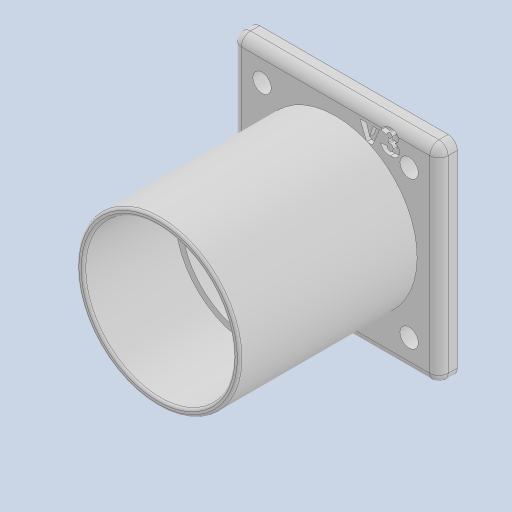
# Autodesk Inventor part: cage_outside_03
Saved by Autodesk Inventor 2024.4 (Build 284460000, 460)
## iProperties
Created: 2026-03-31
Part Number: cage_outside_03
Material: Generic
Document SubType Name: Modeling
Designer: tooles01
Density: 1 g/cm^3
Appearance: Default
Author: tooles01
Autodesk Inventor part; units mm, degrees
ref_plane "YZ Plane" through (0, 0, 0) normal (1, 0, 0) x (0, 1, 0)
ref_plane "XZ Plane" through (0, 0, 0) normal (0, 1, 0) x (-1, 0, 0)
ref_plane "XY Plane" through (0, 0, 0) normal (0, 0, 1) x (1, 0, 0)
sketch "Sketch1: base" plane through (0, 0, 0) normal (0, 0, 1) x (1, 0, 0)
  circle A0 centre (34.5, 31.5) radius 16.25
  line L0 (12, 54) -> (57, 54)
  line L1 (57, 54) -> (57, 9)
  line L2 (57, 9) -> (12, 9)
  line L3 (12, 9) -> (12, 54)
  line L4 (18.5, 47.5) -> (50.5, 47.5) construction
  line L5 (50.5, 47.5) -> (50.5, 15.5) construction
  line L6 (50.5, 15.5) -> (18.5, 15.5) construction
  line L7 (18.5, 15.5) -> (18.5, 47.5) construction
  circle A1 centre (50.5, 47.5) radius 1.8 construction
  circle A2 centre (50.5, 47.5) radius 3.25 construction
  circle A3 centre (34.5, 31.5) radius 17.75
  point P0 (0, 0)
  point P1 (34.5, 54)
  point P2 (12, 31.5)
  point P3 (34.5, 47.5)
  point P4 (50.5, 31.5)
  point P5 (57, 31.5)
  dimension "d0" = 45
  dimension "d1" = 32
  dimension "d2" = 6.5
  dimension "d3" = 3.6
  dimension "d4" = 32.5
  dimension "d6" = 6.5
  dimension "d18" = 1.5
  constraints: 16 end point, 7 perpendicular, 5 midpoint, 4 centre point, 3 coincident, 2 horizontal, 2 horizontal alignment, 2 vertical alignment, 1 other
  measures "d0" distance of L0.start L0.end
  measures "d1" distance of L4.start L4.end
  measures "d2" diameter of A2
  measures "d3" diameter of A1
  measures "d4" diameter of A0
  measures "d6" distance between parallel lines of L1 L5
  measures "d18" radial gap between concentric circles of A3 A0
extrude "Ex1: base" add sketch "Sketch1: base" along normal blind 4 contours L0 L1 L2 L3
sketch "Sketch2: tube stopper" plane through (0, 0, 0) normal (0, 0, 1) x (1, 0, 0)
  circle A0 centre (34.5, 31.5) radius 14.875
  circle A1 centre (34.5, 31.5) radius 16.25 projected
  point P0 (0, 0)
  dimension "d22" = 29.75
  constraints: 1 centre point, 1 coincident
  measures "d22" diameter of A0
hole "Hole1: M3 inserts" at (18.5, 47.5, 0) at (18.5, 15.5, 0) at (50.5, 15.5, 0) at (50.5, 47.5, 0) direction (0, 0, 1) diameter 4 end through all
extrude "Ex2: tube cover" add sketch "Sketch1: base" along normal blind 42.6 contours A3
extrude "Ex3: tube stopper" add sketch "Sketch2: tube stopper" along normal blind 22.6
fillet "Fillet1: outside edges" radius 2 8 edges at (34.5, 54, 4) (57, 54, 2) (57, 31.5, 4) (57, 9, 2) (34.5, 9, 4) (12, 31.5, 4) (12, 54, 2) (12, 9, 2)
fillet "Fillet2: tube cover" radius 0.5 2 edges at (18.25, 31.5, 42.6) (16.75, 31.5, 42.6)
fillet "Fillet3: heat-set" radius 0.75 4 edges at (18.5, 13.5, 0) (50.5, 13.5, 0) (18.5, 45.5, 0) (50.5, 45.5, 0)
sketch "Sketch4: text" plane through (0, 0, 0) normal (0, 0, 1) x (1, 0, 0)
  line L0 (42.5, 52) -> (46, 52) construction
  line L1 (46, 52) -> (46, 48.5) construction
  line L2 (46, 48.5) -> (42.5, 48.5) construction
  line L3 (42.5, 48.5) -> (42.5, 52) construction
  line L4 (12, 54) -> (57, 54) construction
  line L5 (39.7938, 51.3737) -> (41.2375, 51.3737)
  line L6 (41.2375, 51.3737) -> (41.9449, 49.0782)
  line L7 (41.9449, 49.0782) -> (42.6716, 51.3737)
  line L8 (42.6716, 51.3737) -> (44.0719, 51.3737)
  line L9 (44.0719, 51.3737) -> (42.532, 47.75)
  line L10 (42.532, 47.75) -> (41.3, 47.75)
  line L11 (41.3, 47.75) -> (39.7938, 51.3737)
  line L12 (45.6889, 51.3063) -> (44.3751, 51.5421)
  spline S0 degree 2 poles (44.3751, 51.5421) (44.5387, 52.1677) (45.4675, 52.8366) (46.3193, 52.8366) knots 0 0 0 1 2 2 2
  spline S1 degree 2 poles (46.3193, 52.8366) (47.301, 52.8366) (48.172, 52.1051) (48.172, 51.5565) knots 0 0 0 1 2 2 2
  spline S2 degree 2 poles (48.172, 51.5565) (48.172, 51.2293) (47.8159, 50.7048) (47.455, 50.5075) knots 0 0 0 1 2 2 2
  spline S3 degree 2 poles (47.455, 50.5075) (47.7486, 50.4353) (47.9026, 50.339) knots 0 0 0 1 1 1
  spline S4 degree 2 poles (47.9026, 50.339) (48.1528, 50.185) (48.4271, 49.6846) (48.4271, 49.3381) knots 0 0 0 1 2 2 2
  spline S5 degree 2 poles (48.4271, 49.3381) (48.4271, 48.9001) (47.9699, 48.0965) (47.1133, 47.6634) (46.4107, 47.6634) knots 0 0 0 1 2 3 3 3
  spline S6 degree 2 poles (46.4107, 47.6634) (45.7322, 47.6634) (44.943, 47.9858) (44.4329, 48.6018) (44.2981, 49.0686) knots 0 0 0 1 2 3 3 3
  line L13 (44.2981, 49.0686) -> (45.6889, 49.2514)
  spline S7 degree 2 poles (45.6889, 49.2514) (45.7707, 48.8328) (46.1124, 48.5103) (46.377, 48.5103) knots 0 0 0 1 2 2 2
  spline S8 degree 2 poles (46.377, 48.5103) (46.6562, 48.5103) (47.0267, 48.9194) (47.0267, 49.2611) knots 0 0 0 1 2 2 2
  spline S9 degree 2 poles (47.0267, 49.2611) (47.0267, 49.6124) (46.6706, 49.9925) (46.3626, 49.9925) knots 0 0 0 1 2 2 2
  spline S10 degree 2 poles (46.3626, 49.9925) (46.199, 49.9925) (45.9151, 49.9107) knots 0 0 0 1 1 1
  line L14 (45.9151, 49.9107) -> (45.9872, 50.9069)
  spline S11 degree 2 poles (45.9872, 50.9069) (46.1027, 50.8876) (46.1653, 50.8876) knots 0 0 0 1 1 1
  spline S12 degree 2 poles (46.1653, 50.8876) (46.4396, 50.8876) (46.8053, 51.2341) (46.8053, 51.4747) knots 0 0 0 1 2 2 2
  spline S13 degree 2 poles (46.8053, 51.4747) (46.8053, 51.7009) (46.531, 51.9752) (46.2952, 51.9752) knots 0 0 0 1 2 2 2
  spline S14 degree 2 poles (46.2952, 51.9752) (46.0498, 51.9752) (45.7418, 51.6769) (45.6889, 51.3063) knots 0 0 0 1 2 2 2
  point P0 (0, 0)
  point P1 (34.5, 54)
  point P2 (44.25, 52)
  dimension "d26" = 3.5
  dimension "d27" = 2
  dimension "d31" = 11
  constraints: 2 midpoint, 1 horizontal, 1 perpendicular, 2 other
  measures "d26" distance of L0.start L0.end
  measures "d27" distance between parallel lines of L0 L4
  measures "d31" distance from line of L4.end L1
extrude "Ex4: text" cut sketch "Sketch4: text" against normal blind 1 from surface at 4
body "Solid1"
